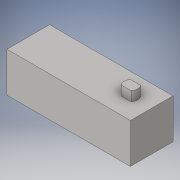
# Autodesk Inventor part: Zoetrope_Motor
Saved by Autodesk Inventor 2016 (Build 200138000, 138)
## iProperties
Created: 2019-01-16
Part Number: Zoetrope_Motor
Material: Generic
Document SubType Name: Modeling
Designer: student
Density: 1 g/cm^3
Appearance: Default
Author: student
Autodesk Inventor part; units mm, degrees
ref_plane "YZ Plane" through (0, 0, 0) normal (1, 0, 0) x (0, 1, 0)
ref_plane "XZ Plane" through (0, 0, 0) normal (0, 1, 0) x (-1, 0, 0)
ref_plane "XY Plane" through (0, 0, 0) normal (0, 0, 1) x (1, 0, 0)
sketch "Sketch1" plane through (0, 0, 0) normal (0, 0, 1) x (1, 0, 0)
  line L0 (0, 0) -> (65.405, 0)
  line L1 (65.405, 0) -> (65.405, 21.082)
  line L2 (65.405, 21.082) -> (0, 21.082)
  line L3 (0, 21.082) -> (0, 0)
  dimension "d0" = 65.405
  dimension "d1" = 21.082
  constraints: 8 end point, 2 parallel, 1 horizontal, 1 perpendicular
  measures "d0" distance of L2.end L1.end
  measures "d1" distance of L1.end L0.end
extrude "Extrusion1" add sketch "Sketch1" along normal blind 22.606
sketch "Sketch2" plane through (0, 21.082, 0) normal (0, 1, 0) x (1, 0, 0)
  line L0 (65.405, 0) -> (65.405, -22.606) projected
  line L1 (65.405, -11.303) -> (54.356, -11.303)
  line L2 (57.023, -8.8265) -> (51.689, -8.8265)
  line L3 (51.689, -13.7795) -> (57.023, -13.7795)
  line L4 (57.023, -8.8265) -> (51.689, -13.7795) construction
  line L5 (51.689, -8.8265) -> (57.023, -13.7795) construction
  arc A0 (51.689, -8.8265) -> (51.689, -13.7795) centre (54.6939, -11.303) ccw
  arc A1 (57.023, -13.7795) -> (57.023, -8.8265) centre (54.0181, -11.303) ccw
  point P0 (0, 0)
  dimension "d4" = 11.049
  dimension "d5" = 5.334
  constraints: 10 end point, 4 point on circle, 3 midpoint, 2 centre point, 2 horizontal, 1 parallel
  measures "d4" distance of L1.start L1.end
  measures "d5" distance of L3.end L3.start
extrude "Extrusion2" add sketch "Sketch2" along normal blind 5.08
body "Solid1"
